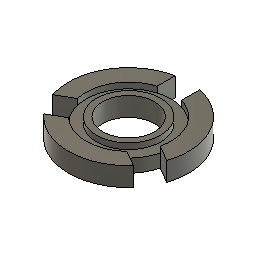
Encaixe v1 (Autodesk Fusion 360 design; units mm, degrees)
Autodesk Fusion 360 part; units mm, degrees
sketch "Esboço1" plane through (0, 0, 0) normal (0, 1, 0) x (1, 0, 0)
  circle A0 centre (0, 0) radius 13.3
  circle A1 centre (0, 0) radius 9.4
  circle A2 centre (0, 0) radius 7.1
  circle A3 centre (0, 0) radius 5.75
  line L0 (-2.7, 13.0231) -> (-2.7, 9.0039)
  line L1 (2.7, 9.0039) -> (2.7, 13.0231)
  line L2 (0, 0) -> (0, 16.7513) construction
  line L3 (-9.9283, -8.8498) -> (-6.4476, -6.8402)
  line L4 (-9.1476, -2.1637) -> (-12.6283, -4.1733)
  line L5 (12.6283, -4.1733) -> (9.1476, -2.1637)
  line L6 (6.4476, -6.8402) -> (9.9283, -8.8498)
  dimension "d1" = 11.5
  dimension "d2" = 14.2
  dimension "d3" = 18.8
  dimension "d4" = 26.6
  dimension "d5" = 5.4
  dimension "d6" = 2.7
  dimension "d8" = 360
  constraint coincident A0.centre A1.centre
  constraint concentric A1 A2
  constraint concentric A2 A3
  constraint coincident A0 L0.start
  constraint coincident A1 L0.end
  constraint vertical L0
  constraint coincident A1 L1.start
  constraint coincident A0 L1.end
  constraint parallel L0 L1
  constraint vertical L2
  measures "d1" diameter of A3
  measures "d2" diameter of A2
  measures "d3" diameter of A1
  measures "d4" diameter of A0
  measures "d5" distance of L0 L1
  measures "d6" distance of L0 L2
extrude "Extrusão1" add sketch "Esboço1" along normal blind 4.2 contours A0 A1 L1 L5 | A0 A1 L0 L4 | A0 A1 L3 L6 | A2 makes body 1 at (12.9632, 2.8, 2.9742) makes body 2 at (7.0647, 1.4, 0.7069) makes body 3 at (6.551, 2.8, 11.5747) makes body 4 at (-12.8098, 2.8, 3.5776)
extrude "Extrusão2" add sketch "Esboço1" along normal blind 2.9 contours A1 bodies 1 2 3 4
